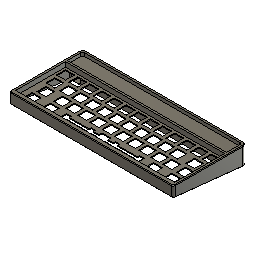
13u Case v2 (Autodesk Fusion 360 design; units mm, degrees)
Autodesk Fusion 360 part; units mm, degrees
sketch "13uswitchplate" plane through (0, 0, 0) normal (0, 1, 0) x (1, 0, 0)
  line L0 (63.3938, 9.2838) -> (63.3938, 3.0138)
  line L1 (0.0951, 0.2577) -> (0.0951, 76.4575)
  line L2 (62.5697, 9.2838) -> (63.3938, 9.2838)
  line L3 (68.4195, 1.8135) -> (68.4195, 3.0138)
  line L4 (101.494, 3.0138) -> (103.219, 3.0138)
  line L5 (63.3938, 12.0826) -> (62.5697, 12.0826)
  line L6 (70.1449, 7.4827) -> (70.6395, 7.4827)
  line L7 (108.245, 15.3128) -> (101.494, 15.3128)
  line L8 (70.1449, 3.0138) -> (70.1449, 7.4827)
  line L9 (65.1192, 3.0138) -> (65.1192, 1.8135)
  line L10 (77.3892, 7.4827) -> (101.494, 7.4827)
  line L11 (63.3938, 3.0138) -> (65.1192, 3.0138)
  line L12 (101.494, 12.0826) -> (77.3892, 12.0826)
  line L13 (101.494, 7.4827) -> (101.494, 3.0138)
  line L14 (121.682, 40.8838) -> (121.682, 54.8831)
  line L15 (116.632, 54.8831) -> (116.632, 40.8838)
  line L16 (116.632, 40.8838) -> (102.632, 40.8838)
  line L17 (102.632, 54.8831) -> (116.632, 54.8831)
  line L18 (65.1192, 1.8135) -> (68.4195, 1.8135)
  line L19 (102.632, 40.8838) -> (102.632, 54.8831)
  line L20 (135.682, 40.8838) -> (121.682, 40.8838)
  line L21 (62.5697, 12.0826) -> (62.5697, 9.2838)
  line L22 (70.6395, 12.0826) -> (70.1449, 12.0826)
  line L23 (228.837, 35.833) -> (242.838, 35.833)
  line L24 (247.745, 0.2577) -> (0.0951, 0.2577)
  line L25 (108.245, 12.0826) -> (108.245, 15.3128)
  line L26 (177.694, 7.4827) -> (177.694, 3.0138)
  line L27 (108.245, 3.0138) -> (108.245, 7.4827)
  line L28 (146.345, 7.4827) -> (170.64, 7.4827)
  line L29 (179.419, 1.8135) -> (182.719, 1.8135)
  line L30 (103.219, 3.0138) -> (103.219, 1.8135)
  line L31 (146.345, 3.0138) -> (146.345, 7.4827)
  line L32 (228.837, 21.8336) -> (228.837, 35.833)
  line L33 (68.4195, 3.0138) -> (70.1449, 3.0138)
  line L34 (103.219, 1.8135) -> (106.519, 1.8135)
  line L35 (144.619, 3.0138) -> (146.345, 3.0138)
  line L36 (116.92, 12.0826) -> (108.245, 12.0826)
  line L37 (0.0951, 76.4575) -> (247.745, 76.4575)
  line L38 (131.014, 2.7836) -> (131.014, 7.4827)
  line L39 (179.419, 3.0138) -> (179.419, 1.8135)
  line L40 (184.445, 9.2838) -> (185.269, 9.2838)
  line L41 (116.92, 2.7836) -> (131.014, 2.7836)
  line L42 (221.407, 35.833) -> (221.407, 21.8336)
  line L43 (70.1449, 12.0826) -> (70.1449, 15.3128)
  line L44 (106.519, 1.8135) -> (106.519, 3.0138)
  line L45 (116.92, 16.7831) -> (116.92, 12.0826)
  line L46 (184.445, 3.0138) -> (184.445, 9.2838)
  line L47 (141.319, 1.8135) -> (144.619, 1.8135)
  line L48 (182.719, 3.0138) -> (184.445, 3.0138)
  line L49 (185.269, 9.2838) -> (185.269, 12.0826)
  line L50 (70.1449, 15.3128) -> (63.3938, 15.3128)
  line L51 (139.594, 7.4827) -> (139.594, 3.0138)
  line L52 (131.014, 7.4827) -> (139.594, 7.4827)
  line L53 (131.014, 12.0826) -> (131.014, 16.7831)
  line L54 (108.245, 7.4827) -> (116.92, 7.4827)
  line L55 (144.619, 1.8135) -> (144.619, 3.0138)
  line L56 (139.594, 3.0138) -> (141.319, 3.0138)
  line L57 (177.694, 3.0138) -> (179.419, 3.0138)
  line L58 (101.494, 15.3128) -> (101.494, 12.0826)
  line L59 (141.319, 3.0138) -> (141.319, 1.8135)
  line L60 (106.519, 3.0138) -> (108.245, 3.0138)
  line L61 (247.745, 76.4575) -> (247.745, 0.2577)
  line L62 (63.3938, 15.3128) -> (63.3938, 12.0826)
  line L63 (116.92, 7.4827) -> (116.92, 2.7836)
  line L64 (177.389, 7.4827) -> (177.694, 7.4827)
  line L65 (182.719, 1.8135) -> (182.719, 3.0138)
  line L66 (207.407, 35.833) -> (221.407, 35.833)
  line L67 (242.838, 35.833) -> (242.838, 21.8336)
  line L68 (21.3817, 16.7831) -> (21.3817, 2.7836)
  line L69 (185.269, 12.0826) -> (184.445, 12.0826)
  line L70 (170.64, 12.0826) -> (146.345, 12.0826)
  line L71 (126.157, 35.833) -> (126.157, 21.8336)
  line L72 (183.307, 35.833) -> (183.307, 21.8336)
  line L73 (150.257, 21.8336) -> (150.257, 35.833)
  line L74 (35.9572, 2.7836) -> (35.9572, 16.7831)
  line L75 (139.594, 12.0826) -> (131.014, 12.0826)
  line L76 (7.3822, 2.7836) -> (7.3822, 16.7831)
  line L77 (164.257, 35.833) -> (164.257, 21.8336)
  line L78 (184.445, 12.0826) -> (184.445, 15.3128)
  line L79 (159.782, 54.8831) -> (173.782, 54.8831)
  line L80 (131.014, 16.7831) -> (116.92, 16.7831)
  line L81 (183.307, 21.8336) -> (169.307, 21.8336)
  line L82 (107.107, 35.833) -> (107.107, 21.8336)
  line L83 (177.694, 12.0826) -> (177.389, 12.0826)
  line L84 (169.307, 35.833) -> (183.307, 35.833)
  line L85 (173.782, 54.8831) -> (173.782, 40.8838)
  line L86 (197.882, 16.7831) -> (211.882, 16.7831)
  line L87 (145.207, 35.833) -> (145.207, 21.8336)
  line L88 (154.732, 54.8831) -> (154.732, 40.8838)
  line L89 (192.832, 54.8831) -> (192.832, 40.8838)
  line L90 (49.9565, 16.7831) -> (49.9565, 2.7836)
  line L91 (35.9572, 16.7831) -> (49.9565, 16.7831)
  line L92 (240.457, 2.7836) -> (226.457, 2.7836)
  line L93 (49.9565, 2.7836) -> (35.9572, 2.7836)
  line L94 (146.345, 15.3128) -> (139.594, 15.3128)
  line L95 (224.076, 54.8831) -> (238.075, 54.8831)
  line L96 (131.207, 35.833) -> (145.207, 35.833)
  line L97 (202.357, 21.8336) -> (188.357, 21.8336)
  line L98 (69.0065, 35.833) -> (69.0065, 21.8336)
  line L99 (211.882, 2.7836) -> (197.882, 2.7836)
  line L100 (177.694, 15.3128) -> (177.694, 12.0826)
  line L101 (121.682, 54.8831) -> (135.682, 54.8831)
  line L102 (202.357, 35.833) -> (202.357, 21.8336)
  line L103 (21.3817, 2.7836) -> (7.3822, 2.7836)
  line L104 (139.594, 15.3128) -> (139.594, 12.0826)
  line L105 (112.157, 35.833) -> (126.157, 35.833)
  line L106 (7.3822, 16.7831) -> (21.3817, 16.7831)
  line L107 (145.207, 21.8336) -> (131.207, 21.8336)
  line L108 (23.7629, 35.833) -> (23.7629, 21.8336)
  line L109 (242.838, 21.8336) -> (228.837, 21.8336)
  line L110 (146.345, 12.0826) -> (146.345, 15.3128)
  line L111 (164.257, 21.8336) -> (150.257, 21.8336)
  line L112 (93.1072, 35.833) -> (107.107, 35.833)
  line L113 (55.0072, 21.8336) -> (55.0072, 35.833)
  line L114 (240.457, 16.7831) -> (240.457, 2.7836)
  line L115 (112.157, 21.8336) -> (112.157, 35.833)
  line L116 (154.732, 40.8838) -> (140.732, 40.8838)
  line L117 (226.457, 16.7831) -> (240.457, 16.7831)
  line L118 (184.445, 15.3128) -> (177.694, 15.3128)
  line L119 (126.157, 21.8336) -> (112.157, 21.8336)
  line L120 (207.407, 21.8336) -> (207.407, 35.833)
  line L121 (131.207, 21.8336) -> (131.207, 35.833)
  line L122 (221.407, 21.8336) -> (207.407, 21.8336)
  line L123 (211.882, 16.7831) -> (211.882, 2.7836)
  line L124 (150.257, 35.833) -> (164.257, 35.833)
  line L125 (188.357, 35.833) -> (202.357, 35.833)
  line L126 (169.307, 21.8336) -> (169.307, 35.833)
  line L127 (188.357, 21.8336) -> (188.357, 35.833)
  line L128 (197.882, 2.7836) -> (197.882, 16.7831)
  line L129 (226.457, 2.7836) -> (226.457, 16.7831)
  line L130 (5.0009, 54.8831) -> (19.0004, 54.8831)
  line L131 (193.12, 73.9331) -> (207.119, 73.9331)
  line L132 (135.682, 54.8831) -> (135.682, 40.8838)
  line L133 (92.819, 73.9331) -> (92.819, 59.9338)
  line L134 (173.782, 40.8838) -> (159.782, 40.8838)
  line L135 (140.732, 54.8831) -> (154.732, 54.8831)
  line L136 (92.819, 59.9338) -> (78.8197, 59.9338)
  line L137 (59.4815, 54.8831) -> (59.4815, 40.8838)
  line L138 (73.769, 59.9338) -> (59.7697, 59.9338)
  line L139 (35.9572, 35.833) -> (49.9565, 35.833)
  line L140 (238.075, 54.8831) -> (238.075, 40.8838)
  line L141 (192.832, 40.8838) -> (178.832, 40.8838)
  line L142 (130.919, 59.9338) -> (116.918, 59.9338)
  line L143 (83.5822, 54.8831) -> (97.5815, 54.8831)
  line L144 (49.9565, 21.8336) -> (35.9572, 21.8336)
  line L145 (40.4315, 54.8831) -> (40.4315, 40.8838)
  line L146 (169.019, 73.9331) -> (169.019, 59.9338)
  line L147 (224.076, 40.8838) -> (224.076, 54.8831)
  line L148 (97.8683, 59.9338) -> (97.8683, 73.9331)
  line L149 (174.07, 59.9338) -> (174.07, 73.9331)
  line L150 (59.4815, 40.8838) -> (45.4822, 40.8838)
  line L151 (178.832, 40.8838) -> (178.832, 54.8831)
  line L152 (59.7697, 59.9338) -> (59.7697, 73.9331)
  line L153 (74.0572, 21.8336) -> (74.0572, 35.833)
  line L154 (197.882, 54.8831) -> (211.882, 54.8831)
  line L155 (69.0065, 21.8336) -> (55.0072, 21.8336)
  line L156 (55.0072, 35.833) -> (69.0065, 35.833)
  line L157 (88.0565, 35.833) -> (88.0565, 21.8336)
  line L158 (78.8197, 59.9338) -> (78.8197, 73.9331)
  line L159 (155.02, 59.9338) -> (155.02, 73.9331)
  line L160 (40.7197, 73.9331) -> (54.719, 73.9331)
  line L161 (245.219, 73.9331) -> (245.219, 59.9338)
  line L162 (5.0009, 40.8838) -> (5.0009, 54.8831)
  line L163 (19.0004, 54.8831) -> (19.0004, 40.8838)
  line L164 (59.7697, 73.9331) -> (73.769, 73.9331)
  line L165 (245.219, 59.9338) -> (231.22, 59.9338)
  line L166 (178.832, 54.8831) -> (192.832, 54.8831)
  line L167 (149.969, 73.9331) -> (149.969, 59.9338)
  line L168 (93.1072, 21.8336) -> (93.1072, 35.833)
  line L169 (97.8683, 73.9331) -> (111.869, 73.9331)
  line L170 (73.769, 73.9331) -> (73.769, 59.9338)
  line L171 (188.069, 73.9331) -> (188.069, 59.9338)
  line L172 (197.882, 40.8838) -> (197.882, 54.8831)
  line L173 (169.019, 59.9338) -> (155.02, 59.9338)
  line L174 (135.97, 73.9331) -> (149.969, 73.9331)
  line L175 (140.732, 40.8838) -> (140.732, 54.8831)
  line L176 (9.762, 35.833) -> (23.7629, 35.833)
  line L177 (78.8197, 73.9331) -> (92.819, 73.9331)
  line L178 (212.17, 59.9338) -> (212.17, 73.9331)
  line L179 (226.169, 59.9338) -> (212.17, 59.9338)
  line L180 (97.5815, 54.8831) -> (97.5815, 40.8838)
  line L181 (74.0572, 35.833) -> (88.0565, 35.833)
  line L182 (155.02, 73.9331) -> (169.019, 73.9331)
  line L183 (35.9572, 21.8336) -> (35.9572, 35.833)
  line L184 (211.882, 40.8838) -> (197.882, 40.8838)
  line L185 (49.9565, 35.833) -> (49.9565, 21.8336)
  line L186 (23.7629, 21.8336) -> (9.762, 21.8336)
  line L187 (238.075, 40.8838) -> (224.076, 40.8838)
  line L188 (107.107, 21.8336) -> (93.1072, 21.8336)
  line L189 (159.782, 40.8838) -> (159.782, 54.8831)
  line L190 (9.762, 21.8336) -> (9.762, 35.833)
  line L191 (88.0565, 21.8336) -> (74.0572, 21.8336)
  line L192 (231.22, 59.9338) -> (231.22, 73.9331)
  line L193 (211.882, 54.8831) -> (211.882, 40.8838)
  line L194 (21.6697, 59.9338) -> (21.6697, 73.9331)
  line L195 (45.4822, 40.8838) -> (45.4822, 54.8831)
  line L196 (116.918, 59.9338) -> (116.918, 73.9331)
  line L197 (2.6197, 59.9338) -> (2.6197, 73.9331)
  line L198 (16.6192, 59.9338) -> (2.6196, 59.9338)
  line L199 (188.069, 59.9338) -> (174.07, 59.9338)
  line L200 (40.7197, 59.9338) -> (40.7197, 73.9331)
  line L201 (226.169, 73.9331) -> (226.169, 59.9338)
  line L202 (64.5322, 54.8831) -> (78.5315, 54.8831)
  line L203 (130.919, 73.9331) -> (130.919, 59.9338)
  line L204 (193.12, 59.9338) -> (193.12, 73.9331)
  line L205 (78.5315, 54.8831) -> (78.5315, 40.8838)
  line L206 (83.5822, 40.8838) -> (83.5822, 54.8831)
  line L207 (26.4322, 54.8831) -> (40.4315, 54.8831)
  line L208 (19.0004, 40.8838) -> (5.0009, 40.8838)
  line L209 (116.918, 73.9331) -> (130.919, 73.9331)
  line L210 (16.6192, 73.9331) -> (16.6192, 59.9338)
  line L211 (149.969, 59.9338) -> (135.97, 59.9338)
  line L212 (111.869, 59.9338) -> (97.8683, 59.9338)
  line L213 (54.719, 59.9338) -> (40.7197, 59.9338)
  line L214 (2.6197, 73.9331) -> (16.6192, 73.9331)
  line L215 (26.4322, 40.8838) -> (26.4322, 54.8831)
  line L216 (54.719, 73.9331) -> (54.719, 59.9338)
  line L217 (207.119, 59.9338) -> (193.12, 59.9338)
  line L218 (111.869, 73.9331) -> (111.869, 59.9338)
  line L219 (35.669, 73.9331) -> (35.669, 59.9338)
  line L220 (45.4822, 54.8831) -> (59.4815, 54.8831)
  line L221 (135.97, 59.9338) -> (135.97, 73.9331)
  line L222 (64.5322, 40.8838) -> (64.5322, 54.8831)
  line L223 (174.07, 73.9331) -> (188.069, 73.9331)
  line L224 (35.669, 59.9338) -> (21.6697, 59.9338)
  line L225 (207.119, 73.9331) -> (207.119, 59.9338)
  line L226 (78.5315, 40.8838) -> (64.5322, 40.8838)
  line L227 (231.22, 73.9331) -> (245.219, 73.9331)
  line L228 (40.4315, 40.8838) -> (26.4322, 40.8838)
  line L229 (21.6697, 73.9331) -> (35.669, 73.9331)
  line L230 (212.17, 73.9331) -> (226.169, 73.9331)
  line L231 (97.5815, 40.8838) -> (83.5822, 40.8838)
  line L232 (177.389, 12.0826) -> (170.64, 12.0826)
  line L233 (170.64, 7.4827) -> (177.389, 7.4827)
  line L234 (70.6395, 12.0826) -> (77.3892, 12.0826)
  line L235 (77.3892, 7.4827) -> (70.6395, 7.4827)
  line L236 (0, 0) -> (247.745, 0)
  line L237 (247.745, 0) -> (247.745, 82.4575)
  line L238 (247.745, 82.4575) -> (0, 82.4575)
  line L239 (0, 82.4575) -> (0, 0)
  line L240 (-5, 108.4575) -> (252.745, 108.4575)
  line L241 (252.745, 108.4575) -> (252.745, -7)
  line L242 (252.745, -7) -> (-5, -7)
  line L243 (-5, -7) -> (-5, 108.4575)
  line L244 (-1, -1) -> (248.745, -1)
  line L245 (248.745, -1) -> (248.745, 83.4575)
  line L246 (248.745, 83.4575) -> (-1, 83.4575)
  line L247 (-1, 83.4575) -> (-1, -1)
  line L248 (248.745, -0.7423) -> (-0.9049, -0.7423)
  line L249 (-0.9049, -0.7423) -> (-0.9049, 77.4575)
  line L250 (-0.9049, 77.4575) -> (248.745, 77.4575)
  line L251 (248.745, 77.4575) -> (248.745, -0.7423)
  dimension "d1" = 6
  dimension "d7" = 1
  dimension "d8" = -1
  dimension "d29" = 4
  dimension "d30" = 4
  dimension "d31" = 6
  dimension "d32" = 25
  constraint horizontal L236
  constraint vertical L237
  constraint horizontal L238
  constraint vertical L239
  constraint coincident L236.start L239.end
  constraint collinear L61 L237
  constraint horizontal L240
  constraint vertical L241
  constraint horizontal L242
  constraint vertical L243
  measures "d1" distance of L37 L238
  measures "d29" distance of L243 L247
  measures "d30" distance of L241 L245
  measures "d31" distance of L242 L244
  measures "d32" distance of L240 L246
extrude "Extrude1" add sketch "13uswitchplate" along normal blind 1.4 contours L1 L24 L37 L236 L237 L239 L250 | L1 L24 L37 L61 L237 | L61 L236 L237 L239 L245 L248 L249 L250 L251 | L237 L238 L239 L250 | L237 L238 L239 L244 L245 L246 L247 L248 L249 L250 | L240 L241 L242 L243
extrude "Extrude2" add sketch "13uswitchplate" along normal blind 7.5 from surface at 1.4 contours L237 L238 L239 L250 | L237 L238 L239 L244 L245 L246 L247 L248 L249 L250 | L240 L241 L242 L243
extrude "Extrude3" add sketch "13uswitchplate" against normal blind 20 contours L240 L241 L242 L243
sketch "Sketch2" plane through (-5, 0, 0) normal (-1, 0, 0) x (0, 0, 1)
  line L0 (7, -20) -> (7, 8.9)
  line L1 (7, 8.9) -> (-108.4575, 8.9)
  line L2 (-108.4575, 8.9) -> (-108.4575, -20)
  line L3 (-108.4575, -20) -> (7, -20)
  line L4 (-108.4575, -20) -> (7, -7.8649)
  line L5 (-108.4575, -20) -> (7.5644, -20) construction
  dimension "d16" = 6
  constraint horizontal L5
  constraint coincident L2.end L3.start
  constraint coincident L0 L4.end
  measures "d16" angle of L4 L5
extrude "Extrude4" cut sketch "Sketch2" against normal blind 365 contours L0 L3 L4
sketch "Sketch3" plane through (0, 0, -108.4575) normal (0, 0, -1) x (-1, 0, 0)
  line L0 (5, -20) -> (5, 8.9)
  line L1 (5, 8.9) -> (-252.745, 8.9)
  line L2 (-252.745, 8.9) -> (-252.745, -20)
  line L3 (-252.745, -20) -> (5, -20)
  line L4 (-2.6197, 0) -> (-16.6192, 0)
  line L5 (-16.6192, -3) -> (-2.6196, -3)
  line L6 (-2.6197, -3) -> (-2.6197, -17)
  line L7 (-2.6197, -17) -> (-16.6192, -17)
  line L8 (-16.6192, -17) -> (-16.6192, -3)
  dimension "d19" = 3
  dimension "d20" = 3
  constraint horizontal L5
  constraint vertical L6
  constraint horizontal L7
  constraint vertical L8
  constraint collinear L4.end L5.start L7.end
  constraint collinear L4.start L6.start L6.end
  measures "d19" distance of L4 L5
  measures "d20" distance of L3 L7
extrude "Extrude5" cut sketch "Sketch3" against normal blind 45 contours L5 L6 L7 L8
fillet "Fillet1" radius 3 4 edges at (16.6192, -3, -95.9575) (2.6197, -17, -95.9575) (16.6192, -17, -95.9575) (2.6197, -3, -95.9575)
fillet "Fillet2" radius 3 2 edges at (-5, 0.5175, 7) (252.745, 0.5175, 7)
fillet "Fillet3" radius 7 2 edges at (252.745, -5.55, -108.4575) (-5, -5.55, -108.4575)
sketch "Sketch4" plane through (0, 8.9, 0) normal (0, 1, 0) x (-1, 0, 0)
  arc A0 (-2, -108.4575) -> (5, -101.4575) centre (-2, -101.4575) ccw
  line L0 (5, -101.4575) -> (5, 4)
  arc A1 (5, 4) -> (2, 7) centre (2, 4) ccw
  line L1 (2, 7) -> (-249.745, 7)
  arc A2 (-249.745, 7) -> (-252.745, 4) centre (-249.745, 4) ccw
  line L2 (-252.745, 4) -> (-252.745, -101.4575)
  arc A3 (-252.745, -101.4575) -> (-245.745, -108.4575) centre (-245.745, -101.4575) ccw
  line L3 (-245.745, -108.4575) -> (-2, -108.4575)
  line L4 (0.9049, 0.7423) -> (0.9049, -77.4575)
  line L5 (0.9049, -77.4575) -> (-248.745, -77.4575)
  line L6 (-248.745, -77.4575) -> (-248.745, 0.7423)
  line L7 (-248.745, 0.7423) -> (0.9049, 0.7423)
  line L8 (1, -104.4575) -> (-248.745, -104.4575)
  line L9 (-248.745, -104.4575) -> (-248.745, -81.4575)
  line L10 (-248.745, -81.4575) -> (1, -81.4575)
  line L11 (1, -81.4575) -> (1, -104.4575)
  dimension "d33" = 4
  dimension "d34" = 4
  dimension "d37" = 4
  dimension "d38" = 4
  constraint horizontal L8
  constraint vertical L9
  constraint horizontal L10
  constraint vertical L11
  constraint coincident L8.start L11.end
  measures "d33" distance of L5 L10
  measures "d34" distance of L2 L9
  measures "d37" distance of L3 L8
  measures "d38" distance of L0 L11
extrude "Extrude6" cut sketch "Sketch4" against normal blind 5 contours L8 L9 L10 L11
fillet "Fillet4" radius 3 2 edges at (-1, 6.4, -104.4575) (248.745, 6.4, -104.4575)
chamfer "Chamfer1" distance 1 angle 45 25 edges at (9.6194, -17, -108.4575) (15.7405, -16.1213, -108.4575) (16.6192, -10, -108.4575) (15.7405, -3.8787, -108.4575) (9.6194, -3, -108.4575) (3.4983, -3.8787, -108.4575) (2.6197, -10, -108.4575) (3.4983, -16.1213, -108.4575) (123.8725, 8.9, -81.4575) (-5, 8.9, -48.7287) (-4.1213, 8.9, 6.1213) (123.8725, 8.9, 7) (251.8663, 8.9, 6.1213) (252.745, 8.9, -48.7287) (250.6947, 8.9, -106.4072) (123.8725, 8.9, -108.4575) (-2.9497, 8.9, -106.4072) (-5, -13.7223, -48.7287) (-4.1213, -7.9573, 6.1213) (123.8725, -7.8649, 7) (251.8663, -7.9573, 6.1213) (252.745, -13.7223, -48.7287) (250.6947, -19.7845, -106.4072) (123.8725, -20, -108.4575) (-2.9497, -19.7845, -106.4072)
named bodies: "13U_Case"
